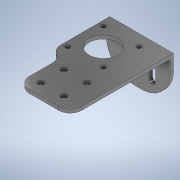
# Autodesk Inventor part: ActuatorPulleyPlate
Saved by Autodesk Inventor 2020.4 (Build 244396010, 396A)
## iProperties
Created: 2021-08-04
Part Number: ActuatorPulleyPlate
Material: Aluminum 6061
Document SubType Name: Modeling
Designer: justi
Density: 2.7 g/cm^3
Appearance: Honed - Dark Gray
Author: justi
Autodesk Inventor part; units mm, degrees
ref_plane "YZ Plane" through (0, 0, 0) normal (1, 0, 0) x (0, 1, 0)
ref_plane "XZ Plane" through (0, 0, 0) normal (0, 1, 0) x (-1, 0, 0)
ref_plane "XY Plane" through (0, 0, 0) normal (0, 0, 1) x (1, 0, 0)
sketch "Sketch1" plane through (0, 0, 0) normal (0, 1, 0) x (-1, 0, 0)
  line L0 (25, 40) -> (-30.5, 40)
  line L1 (-30.5, 40) -> (-30.5, -50)
  line L2 (-30.5, -50) -> (25, -50)
  line L3 (25, -50) -> (25, 40)
  line L4 (25, 40) -> (15, 40)
  line L5 (15, 40) -> (15, 0)
  line L6 (25, -50) -> (25, -40) construction
  line L7 (25, -40) -> (20.5, -40) construction
  line L8 (20.5, -40) -> (20.5, -9) construction
  line L9 (20.5, -9) -> (-10.5, -9) construction
  line L10 (-10.5, -9) -> (-10.5, -40) construction
  line L11 (-10.5, -40) -> (20.5, -40) construction
  circle A0 centre (5, -24.5) radius 12.5
  circle A1 centre (20.5, -9) radius 2
  circle A2 centre (20.5, -40) radius 2
  circle A3 centre (-10.5, -9) radius 2
  circle A4 centre (-10.5, -40) radius 2
  line L12 (15, 40) -> (5, 40) construction
  line L13 (5, 40) -> (5, 30) construction
  line L14 (5, 30) -> (15, 30) construction
  line L15 (15, 30) -> (15, 40) construction
  line L16 (5, 30) -> (-15, 30) construction
  line L17 (-15, 30) -> (-15, 10) construction
  line L18 (-15, 10) -> (5, 10) construction
  line L19 (5, 10) -> (5, 30) construction
  circle A5 centre (5, 30) radius 2.5
  circle A6 centre (5, 10) radius 2.5
  circle A7 centre (-15, 30) radius 2.5
  circle A8 centre (-15, 10) radius 2.5
  line L20 (15, 0) -> (25, 0)
  point P0 (25, -5)
  dimension "d0" = 55.5
  dimension "d1" = 90
  dimension "d2" = 10
  dimension "d3" = 40
  dimension "d4" = 10
  dimension "d5" = 4.5
  dimension "d6" = 31
  dimension "d7" = 31
  dimension "d8" = 31
  dimension "d9" = 25
  dimension "d10" = 4
  dimension "d11" = 4
  dimension "d12" = 4
  dimension "d13" = 4
  dimension "d14" = 10
  dimension "d15" = 10
  dimension "d16" = 20
  dimension "d17" = 20
  dimension "d18" = 5
  dimension "d19" = 5
  dimension "d20" = 5
  dimension "d21" = 5
  dimension "d25" = 15.5
  constraints: 42 end point, 17 coincident, 9 centre point, 9 perpendicular, 6 parallel, 3 horizontal, 3 point on line, 1 midpoint
  measures "d0" distance of L2.end L1.end
  measures "d1" distance of L1.end L0.end
  measures "d2" distance of L0.start L4.end
  measures "d3" distance of L4.end L5.end
  measures "d4" distance of L2.end L6.end
  measures "d5" distance of L6.end L7.end
  measures "d6" distance of L7.end L8.end
  measures "d7" distance of L8.end L9.end
  measures "d8" distance of L9.end L10.end
  measures "d9" diameter of A0
  measures "d10" diameter of A1
  measures "d11" diameter of A2
  measures "d12" diameter of A3
  measures "d13" diameter of A4
  measures "d14" distance of L14.end L13.end
  measures "d15" distance of L13.end L12.end
  measures "d16" distance of L18.end L17.end
  measures "d17" distance of L17.end L16.end
  measures "d18" diameter of A5
  measures "d19" diameter of A6
  measures "d20" diameter of A7
  measures "d21" diameter of A8
  measures "d25" distance from line of L9 A0.centre
extrude "Extrusion1" add sketch "Sketch1" along normal blind 3 contours L5 L20 L3 L2 L1 L0
sketch "Sketch2" plane through (0, 0, 0) normal (0, -1, 0) x (1, 0, 0)
  line L0 (30.5, 40) -> (30.5, -50) projected
  line L1 (-25, -50) -> (-25, 0) projected
  line L2 (30.5, -50) -> (-25, -50)
  line L3 (-25, -50) -> (-25, -47)
  line L4 (-25, -47) -> (30.5, -47)
  line L5 (30.5, -47) -> (30.5, -50)
  point P0 (0, 0)
  dimension "d26" = 3
  constraints: 8 end point, 2 parallel, 1 horizontal, 1 perpendicular, 1 point on line
  measures "d26" distance of L2.end L3.end
extrude "Extrusion2" add sketch "Sketch2" along normal blind 35
sketch "Sketch3" plane through (-25, 0, -47) normal (0, 0, 1) x (1, 0, 0)
  line L0 (55.5, -35) -> (55.5, 3) construction
  line L1 (0, 0) -> (0, -35) projected
  line L2 (10, 3) -> (55.5, 3) construction
  line L3 (55.5, 3) -> (55.5, -17.5) construction
  line L4 (55.5, -17.5) -> (0, -17.5) construction
  line L5 (0, 3) -> (0, -35) construction
  line L6 (55.5, -17.5) -> (40, -17.5) construction
  line L7 (40, -17.5) -> (19.5, -17.5) construction
  line L8 (19.5, -23.5) -> (19.5, -11.5) construction
  line L9 (22.25, -23.5) -> (22.25, -11.5)
  line L10 (16.75, -11.5) -> (16.75, -23.5)
  arc A0 (16.75, -23.5) -> (22.25, -23.5) centre (19.5, -23.5) ccw
  arc A1 (22.25, -11.5) -> (16.75, -11.5) centre (19.5, -11.5) ccw
  line L11 (40, -23.5) -> (40, -11.5) construction
  line L12 (42.75, -23.5) -> (42.75, -11.5)
  line L13 (37.25, -11.5) -> (37.25, -23.5)
  arc A2 (37.25, -23.5) -> (42.75, -23.5) centre (40, -23.5) ccw
  arc A3 (42.75, -11.5) -> (37.25, -11.5) centre (40, -11.5) ccw
  line L14 (10, 0) -> (55.5, 0) projected
  point P0 (25, 0)
  dimension "d38" = 15.5
  dimension "d39" = 20.5
  dimension "d40" = 6
  dimension "d41" = 5.5
  dimension "d42" = 6
  dimension "d43" = 5.5
  dimension "d47" = 17.5
  constraints: 24 end point, 8 point on circle, 8 tangent, 4 centre point, 4 point on line, 3 parallel, 2 midpoint, 1 perpendicular, 1 vertical
  measures "d38" distance of L3.end L6.end
  measures "d39" distance of L6.end L7.end
  measures "d40" distance of L7.end L8.end
  measures "d41" diameter of A1
  measures "d42" distance of L6.end L11.end
  measures "d43" diameter of A3
  measures "d47" distance from line of L14 L7.end
extrude "Extrusion3" cut sketch "Sketch3" against normal through all
fillet "Fillet3" radius 10 4 edges at (-25, 1.5, 0) (-15, 1.5, 40) (30.5, 1.5, 40) (-15, 1.5, 0)
fillet "Fillet4" radius 25 2 edges at (-25, -35, -48.5) (30.5, -35, -48.5)
body "Solid1"
